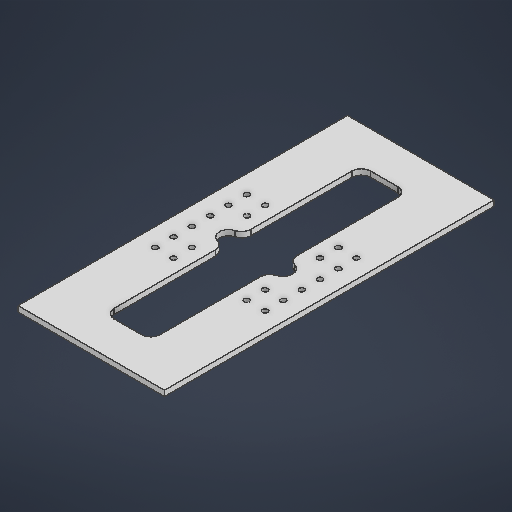
# Autodesk Inventor part: middle_base
Saved by Autodesk Inventor 2026.1 (Build 301233000, 233)
## iProperties
Created: 2026-03-10
Part Number: middle_base
Material: Generic
Document SubType Name: Modeling
Designer: emanuel
Density: 1 g/cm^3
Appearance: Default
Author: emanuel
Autodesk Inventor part; units mm, degrees
ref_plane "YZ Plane" through (0, 0, 0) normal (1, 0, 0) x (0, 1, 0)
ref_plane "XZ Plane" through (0, 0, 0) normal (0, 1, 0) x (-1, 0, 0)
ref_plane "XY Plane" through (0, 0, 0) normal (0, 0, 1) x (1, 0, 0)
sketch "Sketch1" plane through (0, 0, 0) normal (0, 1, 0) x (-1, 0, 0)
  line L0 (0, 0) -> (80, 0)
  line L1 (80, 0) -> (80, -180)
  line L2 (80, -180) -> (0, -180)
  line L3 (0, -180) -> (0, 0)
  line L4 (70, -65) -> (10, -65)
  line L5 (10, -65) -> (10, -115)
  line L6 (10, -115) -> (70, -115)
  line L7 (70, -115) -> (70, -65)
  line L8 (70, -65) -> (10, -115) construction
  line L9 (10, -65) -> (70, -115) construction
  line L10 (70, -75) -> (10, -75)
  line L11 (10, -75) -> (10, -105)
  line L12 (10, -105) -> (70, -105)
  line L13 (70, -105) -> (70, -75)
  line L14 (70, -75) -> (10, -105) construction
  line L15 (10, -75) -> (70, -105) construction
  line L16 (10, -85) -> (70, -85)
  line L17 (70, -85) -> (70, -95)
  line L18 (70, -95) -> (10, -95)
  line L19 (10, -95) -> (10, -85)
  line L20 (10, -85) -> (70, -95) construction
  line L21 (70, -85) -> (10, -95) construction
  circle A0 centre (70, -65) radius 1.5
  circle A1 centre (70, -75) radius 1.5
  circle A2 centre (70, -85) radius 1.5
  circle A3 centre (70, -95) radius 1.5
  circle A4 centre (70, -105) radius 1.5
  circle A5 centre (70, -115) radius 1.5
  circle A6 centre (10, -65) radius 1.5
  circle A7 centre (10, -75) radius 1.5
  circle A8 centre (10, -85) radius 1.5
  circle A9 centre (10, -95) radius 1.5
  circle A10 centre (10, -105) radius 1.5
  circle A11 centre (10, -115) radius 1.5
  line L22 (27.5, -20) -> (52.5, -20)
  line L23 (52.5, -20) -> (52.5, -160)
  line L24 (52.5, -160) -> (27.5, -160)
  line L25 (27.5, -160) -> (27.5, -20)
  line L26 (27.5, -20) -> (52.5, -160) construction
  line L27 (52.5, -20) -> (27.5, -160) construction
  line L28 (20, -65) -> (60, -65)
  line L29 (60, -65) -> (60, -115)
  line L30 (60, -115) -> (20, -115)
  line L31 (20, -115) -> (20, -65)
  line L32 (20, -65) -> (60, -115) construction
  line L33 (60, -65) -> (20, -115) construction
  circle A12 centre (60, -65) radius 1.5
  circle A13 centre (60, -115) radius 1.5
  circle A14 centre (20, -65) radius 1.5
  circle A15 centre (20, -115) radius 1.5
  circle A16 centre (60, -75) radius 1.5
  circle A17 centre (20, -75) radius 1.5
  circle A18 centre (60, -105) radius 1.5
  circle A19 centre (20, -105) radius 1.5
  point P0 (40, -90)
  point P1 (40, -90)
  point P2 (40, -90)
  point P3 (60, -85)
  point P4 (60, -95)
  point P5 (52.5, -95)
  point P6 (27.5, -95)
  point P7 (20, -95)
  point P8 (20, -85)
  point P9 (27.5, -85)
  point P10 (52.5, -85)
  dimension "d0" = 80
  dimension "d1" = 180
  dimension "d4" = 60
  dimension "d5" = 50
  dimension "d6" = 60
  dimension "d7" = 30
  dimension "d8" = 60
  dimension "d9" = 10
  dimension "d10" = 3
  dimension "d11" = 3
  dimension "d12" = 3
  dimension "d13" = 3
  dimension "d14" = 3
  dimension "d15" = 3
  dimension "d16" = 3
  dimension "d17" = 3
  dimension "d18" = 3
  dimension "d19" = 3
  dimension "d20" = 3
  dimension "d21" = 3
  dimension "d22" = 25
  dimension "d23" = 140
  dimension "d24" = 40
  dimension "d25" = 3
  dimension "d26" = 3
  dimension "d27" = 3
  dimension "d28" = 3
  dimension "d29" = 3
  dimension "d30" = 3
  dimension "d31" = 3
  dimension "d32" = 3
  constraints: 68 end point, 20 centre point, 12 midpoint, 12 parallel, 9 point on line, 6 horizontal, 6 perpendicular, 2 coincident
  measures "d0" distance of L1.end L2.end
  measures "d1" distance of L0.end L1.end
  measures "d4" distance of L6.end L5.end
  measures "d5" distance of L5.end L4.end
  measures "d6" distance of L12.end L11.end
  measures "d7" distance of L11.end L10.end
  measures "d8" distance of L17.end L18.end
  measures "d9" distance of L16.end L17.end
  measures "d10" diameter of A0
  measures "d11" diameter of A1
  measures "d12" diameter of A2
  measures "d13" diameter of A3
  measures "d14" diameter of A4
  measures "d15" diameter of A5
  measures "d16" diameter of A6
  measures "d17" diameter of A7
  measures "d18" diameter of A8
  measures "d19" diameter of A9
  measures "d20" diameter of A10
  measures "d21" diameter of A11
  measures "d22" distance of L23.end L24.end
  measures "d23" distance of L22.end L23.end
  measures "d24" distance of L29.end L30.end
  measures "d25" diameter of A12
  measures "d26" diameter of A13
  measures "d27" diameter of A14
  measures "d28" diameter of A15
  measures "d29" diameter of A16
  measures "d30" diameter of A17
  measures "d31" diameter of A18
  measures "d32" diameter of A19
extrude "Extrusion1" add sketch "Sketch1" along normal blind 3 contours L0 L1 L2 L3 | L4 A0 L7 A1 L10 A16 L29 A12 | A12 L29 A16 L10 L23 L4 | L25 L10 A17 L31 A14 L4 | L10 A16 L29 L16 L23 | L10 A1 L7 A2 L16 L29 A16 | L25 L16 L31 A17 L10 | A14 L31 A17 L10 A7 L5 A6 L4 | L16 A2 L7 A3 L18 L29 | L18 L29 A18 L12 L23 | L31 L16 A8 L5 A7 L10 A17 | L31 L18 A9 L5 A8 L16 | L25 L12 A19 L31 L18 | L18 A3 L7 A4 L12 A18 L29 | L12 A18 L29 A13 L6 L23 | L31 A19 L12 A10 L5 A9 L18 | L25 L6 A15 L31 A19 L12 | L12 A4 L7 A5 L6 A13 L29 A18 | A19 L31 A15 L6 A11 L5 A10 L12
fillet "Fillet1" radius 5 12 edges at (-52.5, 1.5, -160) (-27.5, 1.5, -160) (-60, 1.5, -95) (-52.5, 1.5, -95) (-60, 1.5, -85) (-52.5, 1.5, -85) (-52.5, 1.5, -20) (-27.5, 1.5, -20) (-27.5, 1.5, -85) (-20, 1.5, -85) (-20, 1.5, -95) (-27.5, 1.5, -95)
body "Solid1"
